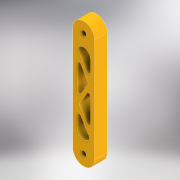
# Autodesk Inventor part: CodoTrasero
Saved by Autodesk Inventor 2021 (Build 250183000, 183)
## iProperties
Created: 2024-02-25
Part Number: CodoTrasero
Material: PLA
Document SubType Name: Modeling
Designer: Martin
Mass: 80.6641 g
Surface Area: 225.37 cm^2
Volume: 63.5151 cm^3
Density: 1.27 g/cm^3
Appearance: PLA
Author: Martin
Autodesk Inventor part; units mm, degrees
ref_plane "YZ Plane" through (0, 0, 0) normal (1, 0, 0) x (0, 1, 0)
ref_plane "XZ Plane" through (0, 0, 0) normal (0, 1, 0) x (-1, 0, 0)
ref_plane "XY Plane" through (0, 0, 0) normal (0, 0, 1) x (1, 0, 0)
sketch "Sketch1" plane through (0, 0, 0) normal (0, 0, 1) x (1, 0, 0)
  line L0 (0, 81.5) -> (0, -81.5) construction
  line L1 (-17, 81.5) -> (-17, -81.5)
  line L2 (17, -81.5) -> (17, 81.5)
  arc A0 (17, 81.5) -> (-17, 81.5) centre (0, 81.5) ccw
  arc A1 (-17, -81.5) -> (17, -81.5) centre (0, -81.5) ccw
  circle A2 centre (0, -81.5) radius 11.075
  circle A3 centre (0, 81.5) radius 11.075
  point P0 (0, 0)
  dimension "d0" = 81.5
  dimension "d1" = 34
  dimension "d2" = 22.15
  dimension "d3" = 22.15
  constraints: 8 end point, 4 centre point, 4 point on circle, 4 tangent, 2 coincident, 1 midpoint, 1 parallel, 1 vertical
  measures "d0" distance of point (0, 0) L0.end
  measures "d1" diameter of A1
  measures "d2" diameter of A2
  measures "d3" diameter of A3
extrude "Extrusion1" add sketch "Sketch1" along normal blind 8
sketch "Sketch2" plane through (0, 0, 8) normal (0, 0, 1) x (1, 0, 0)
  arc A0 (-17, -81.5) -> (17, -81.5) centre (0, -81.5) ccw projected
  line L0 (17, -81.5) -> (17, 81.5) projected
  arc A1 (17, 81.5) -> (-17, 81.5) centre (0, 81.5) ccw projected
  line L1 (-17, 81.5) -> (-17, -81.5) projected
  circle A2 centre (0, 81.5) radius 11.075 projected
  circle A3 centre (0, -81.5) radius 11.075 projected
  circle A4 centre (0, -81.5) radius 4.075
  circle A5 centre (0, 81.5) radius 4.075
  point P0 (0, 0)
  dimension "d6" = 8.15
  dimension "d12" = 8.15
  constraints: 2 centre point, 2 coincident
  measures "d6" diameter of A4
  measures "d12" diameter of A5
extrude "Extrusion2" add sketch "Sketch2" along normal blind 12 contours L1 A1 L0 A0 | A2 | A3
sketch "Sketch3" plane through (0, 0, 20) normal (0, 0, 1) x (1, 0, 0)
  line L0 (17, -81.5) -> (17, 81.5) projected
  arc A0 (17, 81.5) -> (-17, 81.5) centre (0, 81.5) ccw projected
  line L1 (-17, 81.5) -> (-17, -81.5) projected
  arc A1 (-17, -81.5) -> (17, -81.5) centre (0, -81.5) ccw projected
  circle A2 centre (0, -81.5) radius 4.075 projected
  line L2 (0, 52.5) -> (0, -52.5) construction
  line L3 (-10.3409, 52.5) -> (-10.3409, -52.5)
  line L4 (10.3409, -52.5) -> (10.3409, 52.5)
  arc A3 (10.3409, 52.5) -> (-10.3409, 52.5) centre (0, 52.5) ccw
  arc A4 (-10.3409, -52.5) -> (10.3409, -52.5) centre (0, -52.5) ccw
  point P0 (0, -4.7822)
  point P1 (0, 0)
  dimension "d11" = 105
  constraints: 8 end point, 4 point on circle, 4 tangent, 2 centre point, 1 midpoint, 1 parallel, 1 point on line, 1 vertical
  measures "d11" distance of L2.start L2.end
extrude "Extrusion3" cut sketch "Sketch3" against normal up to next contours A3 L4 A4 L3
sketch "Sketch5" plane through (0, 0, 20) normal (0, 0, 1) x (1, 0, 0)
  line L0 (10.3409, 52.5) -> (10.3409, -52.5) projected
  arc A0 (-10.3409, -52.5) -> (10.3409, -52.5) centre (0, -52.5) ccw projected
  line L1 (-10.3409, -52.5) -> (-10.3409, 52.5) projected
  arc A1 (10.3409, 52.5) -> (-10.3409, 52.5) centre (0, 52.5) ccw projected
  line L2 (17, -81.5) -> (17, 81.5) projected
  arc A2 (17, 81.5) -> (-17, 81.5) centre (0, 81.5) ccw projected
  line L3 (-17, 81.5) -> (-17, -81.5) projected
  arc A3 (-17, -81.5) -> (17, -81.5) centre (0, -81.5) ccw projected
  circle A4 centre (0, -81.5) radius 4.075 projected
  circle A5 centre (0, 81.5) radius 4.075 projected
  line L4 (-10.3409, -52.5) -> (-10.3409, -17.5)
  line L5 (-10.3409, 52.5) -> (-10.3409, -52.5) projected
  line L6 (-10.3409, 52.5) -> (-10.3409, 17.5)
  line L7 (10.3409, -52.5) -> (-10.3409, -17.5)
  line L8 (10.3409, 17.5) -> (-10.3409, -17.5)
  line L9 (10.3409, 17.5) -> (-10.3409, 52.5)
  line L10 (9.6433, -56.2337) -> (-12.4932, -18.7718)
  line L11 (12.4932, -51.2282) -> (-8.1886, -16.2282)
  line L12 (-8.1886, -18.7718) -> (13.2448, 17.5)
  line L13 (13.2448, 17.5) -> (-12.8409, 61.645)
  line L14 (-12.8409, 61.645) -> (-12.8409, 17.5)
  line L15 (-12.4932, -16.2282) -> (7.4371, 17.5)
  line L16 (7.4371, 17.5) -> (-10.3409, 47.5858)
  line L17 (-7.8409, 43.355) -> (-7.8409, 17.5)
  point P0 (0, 0)
  point P1 (-7.4371, -17.5)
  point P2 (10.3409, 12.5858)
  point P3 (10.3409, 22.4142)
  point P4 (-9.6433, 56.2337)
  point P5 (-10.3409, -12.5858)
  point P6 (-10.3409, -22.4142)
  point P7 (10.3409, -47.5858)
  dimension "d17" = 35
  dimension "d18" = 35
  dimension "d19" = 2.5
  dimension "d20" = 2.5
  dimension "d21" = 2.5
  dimension "d22" = 2.5
  constraints: 26 end point, 5 point on line, 3 parallel, 1 point on circle, 2 other
  measures "d17" distance of L1.start L4.end
  measures "d18" distance of L1.end L6.end
  measures "d19" distance between parallel lines of L7 L10
  measures "d20" distance between parallel lines of L7 L11
  measures "d21" distance between parallel lines of L8 L12
  measures "d22" distance between parallel lines of L8 L15
extrude "Extrusion5" add sketch "Sketch5" against normal up to surface (20 mm away) contours L0 L9 A1 L13 | L0 L12 L11 L7 L8 | L8 L1 L15 L16 L9 | L7 A0 L10 L1
fillet "Fillet1" radius 3 9 edges at (10.3409, 22.4142, 10) (10.3409, -47.5858, 10) (-7.4371, -17.5, 10) (-10.3409, -22.4142, 10) (7.4371, 17.5, 10) (-10.3409, -12.5858, 10) (-10.3409, 47.5858, 10) (-9.6433, 56.2337, 10) (9.6433, -56.2337, 10)
fillet "Fillet2" radius 3 1 edges at (10.3409, 12.5858, 10)
body "Solid1"
